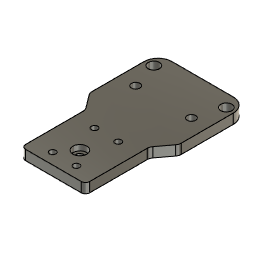
Laser Carriage - Laser Side V2 (Autodesk Fusion 360 design; units mm, degrees)
Autodesk Fusion 360 part; units mm, degrees
note: some values were not read from the file. Set by a fixed rule: which sketch regions a step uses.
sketch "Sketch1" plane through (0, 0, 0) normal (0, 0, 1) x (1, 0, 0) in component "Laser Carriage - Laser Side V2"
  line L0 (0, 0) -> (64, 0)
  line L1 (64, 0) -> (64, 100)
  line L2 (64, 100) -> (0, 100)
  line L3 (0, 100) -> (0, 0)
  dimension "d1" = 64
  dimension "d2" = 100
  constraint horizontal L0
  constraint vertical L1
  constraint horizontal L2
  constraint vertical L3
  constraint coincident L0.start L3.end
  measures "d1" distance of L0.start L0.end
  measures "d2" distance of L0.start L2.end
extrude "Extrude1" add sketch "Sketch1" along normal blind 7 in component "Laser Carriage - Laser Side V2"
sketch "Sketch2" plane through (0, 0, 7) normal (0, 0, 1) x (-1, 0, 0) in component "Laser Carriage - Laser Side V2"
  line L0 (0, -100) -> (0, 0)
  line L1 (0, 0) -> (-64, 0)
  line L2 (-64, 0) -> (-64, -100)
  line L3 (-64, -100) -> (0, -100)
  line L4 (-12, -100) -> (-12, 0) construction
  line L5 (-52, -100) -> (-52, 0) construction
  line L6 (0, -12) -> (-64, -12) construction
  line L7 (0, -72) -> (-64, -72) construction
  circle A0 centre (-12, -72) radius 12 construction
  circle A1 centre (-52, -72) radius 12 construction
  circle A2 centre (-12, -72) radius 3
  circle A3 centre (-52, -72) radius 3
  circle A4 centre (-32, -12) radius 12 construction
  circle A5 centre (-32, -12) radius 2.75
  line L8 (0, -85) -> (-64, -85) construction
  line L9 (-32, -85) -> (-32, 0) construction
  dimension "d8" = 12
  dimension "d13" = 24
  dimension "d14" = 24
  dimension "d16" = 6
  dimension "d17" = 6
  dimension "d40" = 60
  dimension "d54" = 24
  dimension "d56" = 5.5
  dimension "d234" = 13
  dimension "d238" = 20
  dimension "d275" = 20
  constraint coincident L3 L4.start
  constraint coincident L1 L4.end
  constraint perpendicular L1 L4
  constraint coincident L3 L5.start
  constraint coincident L1 L5.end
  constraint perpendicular L1 L5
  constraint coincident L1 L9.end
  constraint coincident L0 L6.start
  constraint coincident L2 L6.end
  constraint perpendicular L2 L6
  constraint coincident L0 L7.start
  constraint coincident L2 L7.end
  constraint perpendicular L2 L7
  constraint coincident L7 A0.centre
  constraint coincident L4 A0.centre
  constraint coincident L7 A1.centre
  constraint coincident L5 A1.centre
  constraint concentric A0 A2
  constraint concentric A1 A3
  constraint coincident L6 A4.centre
  constraint concentric A4 A5
  constraint coincident L0 L8.start
  constraint coincident L2 L8.end
  constraint perpendicular L2 L8
  constraint midpoint L8 L9.start
  constraint midpoint L6 A4.centre
  measures "d8" distance of L1 L6
  measures "d13" diameter of A0
  measures "d14" diameter of A1
  measures "d16" diameter of A2
  measures "d17" diameter of A3
  measures "d40" distance of L6 L7
  measures "d54" diameter of A4
  measures "d56" diameter of A5
  measures "d234" distance of A0.centre L8
  measures "d238" distance of L4 L9
  measures "d275" distance of L5 L9
extrude "Extrude2" cut sketch "Sketch2" against normal up to surface (7 mm away) contours A2 | A3 | A5 in component "Laser Carriage - Laser Side V2"
sketch "Sketch19" plane through (0, 0, 7) normal (0, 0, 1) x (-1, 0, 0) in component "Laser Carriage - Laser Side V2"
  circle A0 centre (-12, -72) radius 3
  circle A1 centre (-52, -72) radius 3
  circle A2 centre (-32, -12) radius 2.75
  line L0 (0, -100) -> (0, 0)
  line L1 (0, 0) -> (-64, 0)
  line L2 (-64, 0) -> (-64, -100)
  line L3 (-64, -100) -> (0, -100)
  line L4 (0, 0) -> (0, 7)
  line L5 (-64, 0) -> (-64, 7)
  line L6 (0, 7) -> (-64, 7)
  dimension "d279" = 7
  dimension "d280" = 7
  constraint coincident L0.end L1.start
  constraint perpendicular L1 L4
  constraint coincident L1.end L2.start
  constraint perpendicular L1 L5
  measures "d279" distance of L0.end L4.end
  measures "d280" distance of L1.end L5.end
extrude "Extrude19" add sketch "Sketch19" against normal blind 7 contours L1 L4 L5 L6 in component "Laser Carriage - Laser Side V2"
fillet "Fillet5" radius 10 2 edges at (0, 100, 3.5) (64, 100, 3.5) in component "Laser Carriage - Laser Side V2"
sketch "Sketch16" plane through (0, 0, 7) normal (0, 0, 1) x (-1, 0, 0) in component "Laser Carriage - Laser Side V2"
  circle A0 centre (-52, -72) radius 3
  circle A1 centre (-12, -72) radius 3
  arc A2 (-64, -90) -> (-54, -100) centre (-54, -90) ccw
  line L0 (-54, -100) -> (-10, -100)
  arc A3 (-10, -100) -> (0, -90) centre (-10, -90) ccw
  line L1 (0, -90) -> (0, 7)
  line L2 (-64, 7) -> (-64, -90)
  line L3 (-32, -100) -> (-32, 0) construction
  line L4 (0, -16) -> (-64, -16) construction
  line L5 (-40.5, -100) -> (-40.5, 0) construction
  line L6 (-23.5, -100) -> (-23.5, 0) construction
  line L7 (0, -31) -> (-64, -31) construction
  line L8 (0, -1) -> (-64, -1) construction
  circle A4 centre (-23.5, -31) radius 2.25
  circle A5 centre (-40.5, -31) radius 2.25
  circle A6 centre (-23.5, -1) radius 2.25
  circle A7 centre (-40.5, -1) radius 2.25
  line L9 (-55, -39) -> (-9, -39)
  line L10 (-9, -39) -> (-9, 7)
  line L11 (-9, 7) -> (-55, 7)
  line L12 (-55, 7) -> (-55, -39)
  line L13 (-55, -39) -> (-9, 7) construction
  line L14 (-9, -39) -> (-55, 7) construction
  circle A8 centre (-32, -12) radius 2.75
  line L15 (0, -91) -> (-64, -91) construction
  line L16 (-64, -100) -> (0, -100) construction
  line L17 (-6, 0) -> (-6, -100) construction
  line L18 (0, -100) -> (0, 0) construction
  line L19 (-58, 0) -> (-58, -100) construction
  circle A9 centre (-6, -91) radius 4
  circle A10 centre (-58, -91) radius 4
  line L20 (0, 0) -> (-64, 0)
  line L21 (0, 7) -> (-64, 7)
  line L22 (0, -51) -> (-64, -51) construction
  line L23 (0, -51) -> (-9, -39)
  line L24 (-64, -51) -> (-55, -39)
  point P0 (-32, -16)
  dimension "d246" = 15
  dimension "d247" = 15
  dimension "d248" = 8.5
  dimension "d249" = 8.5
  dimension "d250" = 4.5
  dimension "d251" = 4.5
  dimension "d252" = 4.5
  dimension "d253" = 4.5
  dimension "d262" = 46
  dimension "d263" = 46
  dimension "d268" = 6
  dimension "d269" = 6
  dimension "d270" = 8
  dimension "d271" = 8
  dimension "d272" = 16
  dimension "d287" = 9
  dimension "d292" = 58
  constraint midpoint L0 L3.start
  constraint coincident L1 L4.start
  constraint perpendicular L3 L4
  constraint coincident L0 L5.start
  constraint coincident L1 L7.start
  constraint coincident L2 L7.end
  constraint perpendicular L2 L7
  constraint coincident L1 L8.start
  constraint coincident L2 L8.end
  constraint perpendicular L2 L8
  constraint coincident L7 A4.centre
  constraint coincident L6 A4.centre
  constraint coincident L7 A5.centre
  constraint coincident L5 A5.centre
  constraint coincident L6 A6.centre
  constraint coincident L8 A6.centre
  constraint coincident L8 A7.centre
  constraint coincident L5 A7.centre
  constraint coincident L2 L4.end
  constraint horizontal L9
  constraint perpendicular L9 L10
  constraint parallel L9 L11
  constraint parallel L10 L12
  constraint coincident L13 P0
  constraint coincident L14 P0
  constraint midpoint L4 P0
  constraint coincident L0 L6.start
  constraint coincident L1 L15.start
  constraint coincident L2 L15.end
  constraint perpendicular L2 L15
  constraint coincident L16 L17.end
  constraint coincident L16 L19.end
  constraint coincident L15 A9.centre
  constraint coincident L17 A9.centre
  constraint coincident L15 A10.centre
  constraint coincident L19 A10.centre
  constraint coincident L1 L22.start
  constraint coincident L2 L22.end
  constraint perpendicular L2 L22
  measures "d246" distance of L4 L7
  measures "d247" distance of L4 L8
  measures "d248" distance of L3 L6
  measures "d249" distance of L3 L5
  measures "d250" diameter of A4
  measures "d251" diameter of A5
  measures "d252" diameter of A6
  measures "d253" diameter of A7
  measures "d262" distance of L10.end L11.end
  measures "d263" distance of L9.end L10.end
  measures "d268" distance of L17 L18
  measures "d269" distance of L2 L19
  measures "d270" diameter of A9
  measures "d271" diameter of A10
  measures "d272" distance of L4 L20
  measures "d287" distance of L0 L15
  measures "d292" distance of L21 L22
extrude "Extrude17" cut sketch "Sketch16" against normal up to surface (7 mm away) contours L2 L12 L20 L24 | L2 L12 L20 L21 | L1 L10 L20 L23 | A7 L20 | A7 L20 | L1 L10 L20 L21 | A6 L20 | A6 L20 | A4 | A5 | A9 | A10 in component "Laser Carriage - Laser Side V2"
sketch "Sketch17" plane through (0, 0, 7) normal (0, 0, 1) x (-1, 0, 0) in component "Laser Carriage - Laser Side V2"
  circle A0 centre (-32, -12) radius 5
  dimension "d276" = 10
  measures "d276" diameter of A0
extrude "Extrude18" cut sketch "Sketch17" against normal blind 4 in component "Laser Carriage - Laser Side V2"
fillet "Fillet13" radius 5 4 edges at (0, 51, 3.5) (9, 39, 3.5) (55, 39, 3.5) (64, 51, 3.5) in component "Laser Carriage - Laser Side V2"
fillet "Fillet13" radius 3 2 edges at (55, -7, 3.5) (9, -7, 3.5) in component "Laser Carriage - Laser Side V2"
component "Laser Carriage - Laser Side V2" placed x (1, 0, 0) y (0, 1, 0) z (0, 0, 1) at (0, 0, 0)
named bodies: "Laser Carriage - Laser Side V2"
